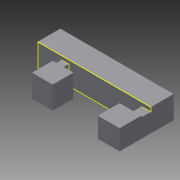
# Autodesk Inventor part: NBS(updated)
Saved by Autodesk Inventor 2013 (Build 170138000, 138)
## iProperties
Created: 2006-04-25
Part Number: NBS(updated)
Document SubType Name: Modeling
Designer: mcgratta
Material: Generic
Density: 1 g/cm^3
Author: mcgratta
Autodesk Inventor part; units mm, degrees
ref_plane "YZ Plane" through (0, 0, 0) normal (1, 0, 0) x (0, 1, 0)
ref_plane "XZ Plane" through (0, 0, 0) normal (0, 1, 0) x (-1, 0, 0)
ref_plane "XY Plane" through (0, 0, 0) normal (0, 0, 1) x (1, 0, 0)
sketch "Sketch1" plane through (0, 0, 0) normal (0, 0, 1) x (1, 0, 0)
  line L0 (-45.8384, 19.9204) -> (12144.1616, 19.9204)
  line L1 (12144.1616, 19.9204) -> (12144.1616, -2420.0796)
  line L2 (12144.1616, -2420.0796) -> (-45.8384, -2420.0796)
  line L3 (-45.8384, -2420.0796) -> (-45.8384, 19.9204)
  line L4 (12144.1616, -2420.0796) -> (11124.1616, -2420.0796)
  line L5 (11124.1616, -2420.0796) -> (11124.1616, -3450.0796)
  line L6 (11124.1616, -3450.0796) -> (12144.1616, -3450.0796)
  line L7 (12144.1616, -3450.0796) -> (12144.1616, -2420.0796)
  line L8 (12144.1616, -3450.0796) -> (9804.1616, -3450.0796)
  line L9 (9804.1616, -3450.0796) -> (9804.1616, -5790.0796)
  line L10 (9804.1616, -5790.0796) -> (12144.1616, -5790.0796)
  line L11 (12144.1616, -5790.0796) -> (12144.1616, -3450.0796)
  line L12 (2525.1057, -2420.0796) -> (3315.1057, -2420.0796)
  line L13 (3315.1057, -2420.0796) -> (3315.1057, -3360.0796)
  line L14 (3315.1057, -3360.0796) -> (2525.1057, -3360.0796)
  line L15 (2525.1057, -3360.0796) -> (2525.1057, -2420.0796)
  line L16 (2525.1057, -3360.0796) -> (4745.1057, -3360.0796)
  line L17 (4745.1057, -3360.0796) -> (4745.1057, -5600.0796)
  line L18 (4745.1057, -5600.0796) -> (2525.1057, -5600.0796)
  line L19 (2525.1057, -5600.0796) -> (2525.1057, -3360.0796)
  dimension "d0" = 12190
  dimension "d1" = 2440
  dimension "d2" = 1020
  dimension "d3" = 1030
  dimension "d4" = 2340
  dimension "d5" = 2340
  dimension "d6" = 940
  dimension "d7" = 790
  dimension "d8" = 2240
  dimension "d9" = 2220
  constraints: 40 end point, 10 parallel, 5 horizontal, 5 perpendicular, 1 point on line
  measures "d0" distance of L0.start L0.end
  measures "d1" distance of L2.end L0.start
  measures "d2" distance of L5.end L6.end
  measures "d3" distance of L6.end L1.end
  measures "d4" distance of L8.end L9.end
  measures "d5" distance of L9.end L10.end
  measures "d6" distance of L12.end L13.end
  measures "d7" distance of L13.end L14.end
  measures "d8" distance of L16.end L17.end
  measures "d9" distance of L17.end L18.end
extrude "Extrusion1" add sketch "Sketch1" along normal blind 2430 contours L14 L16 L17 L18 L19
extrude "Extrusion2" add sketch "Sketch1" along normal blind 2440 contours L0 L1 L2 L3
extrude "Extrusion3" add sketch "Sketch1" along normal blind 2000 contours L7 L6 L5 L2
extrude "Extrusion4" add sketch "Sketch1" along normal blind 2160 contours L11 L10 L9 L8 L6
extrude "Extrusion5" add sketch "Sketch1" along normal blind 2040 contours L2 L13 L14 L15
shell "Shell1" thickness 1 removed faces 0
sketch "Sketch2" plane through (-45.8384, -2420.0796, 0) normal (-1, 0, 0) x (0, 0, 1)
  line L0 (2440, 0) -> (2440, 2440) projected
  line L1 (0, 2440) -> (2440, 2440) projected
  line L2 (0, 2440) -> (0, 0) projected
  line L3 (1, 2439) -> (2439, 2439) projected
sketch "Sketch3" plane through (-45.8384, -2420.0796, 0) normal (-1, 0, 0) x (0, 0, 1)
  line L0 (0, 2440) -> (0, 0) projected
  line L1 (0, 1599) -> (2030, 1599)
  line L2 (2030, 1599) -> (2030, 839)
  line L3 (2030, 839) -> (0, 839)
  line L4 (0, 839) -> (0, 1599)
  line L5 (1, 2439) -> (2439, 2439) projected
  dimension "d25" = 2030
  dimension "d26" = 760
  dimension "d27" = 840
  constraints: 8 end point, 2 parallel, 1 horizontal, 1 perpendicular, 1 point on line
  measures "d25" distance of L1.start L1.end
  measures "d26" distance of L1.end L2.end
  measures "d27" distance between parallel lines of L1 L5
extrude "Extrusion6" cut sketch "Sketch3" against normal mid plane 2
sketch "Sketch4" plane through (-45.8384, -2420.0796, 0) normal (0, -1, 0) x (1, 0, 0)
  line L0 (2570.9442, 0) -> (2570.9442, 2040) projected
  line L1 (2570.9442, 2040) -> (3360.9442, 2040) projected
  line L2 (3360.9442, 2040) -> (3360.9442, 0) projected
  line L3 (3360.9442, 0) -> (11170, 0) projected
  line L4 (11170, 0) -> (11170, 2000) projected
  line L5 (11170, 2000) -> (12190, 2000) projected
  line L6 (12190, 2000) -> (12190, 2440) projected
  line L7 (12190, 2440) -> (0, 2440) projected
  line L8 (0, 0) -> (0, 2440) projected
  line L9 (0, 0) -> (2570.9442, 0) projected
sketch "Sketch5" plane through (9804.1616, -5790.0796, 0) normal (0, -1, 0) x (1, 0, 0)
  line L0 (0, 0) -> (0, 2160) projected
  line L1 (0, 0) -> (2340, 0) projected
  line L2 (1000, 500) -> (1340, 500)
  line L3 (1340, 500) -> (1340, 400)
  line L4 (1340, 400) -> (1000, 400)
  line L5 (1000, 400) -> (1000, 500)
  dimension "d30" = 1000
  dimension "d31" = 340
  dimension "d32" = 100
  dimension "d33" = 500
  constraints: 8 end point, 2 parallel, 1 horizontal, 1 perpendicular
  measures "d30" distance between parallel lines of L5 L0
  measures "d31" distance of L2.start L2.end
  measures "d32" distance of L2.end L3.end
  measures "d33" distance between parallel lines of L1 L2
extrude "Extrusion7" add sketch "Sketch5" against normal blind 340
sketch "Sketch6" plane through (-45.8384, 19.9204, 0) normal (0, 1, 0) x (1, 0, 0)
  line L0 (12190, 0) -> (0, 0) projected
  line L1 (11280, 0) -> (12090, 0)
  constraints: 2 end point, 1 horizontal, 1 point on line
sketch "Sketch7" plane through (-45.8384, 19.9204, 0) normal (0, 1, 0) x (1, 0, 0)
  line L0 (12190, 0) -> (12190, -2440) projected
  line L1 (12190, 0) -> (0, 0) projected
  line L2 (11280, -5) -> (12090, -5)
  line L3 (12090, -5) -> (12090, -1605)
  line L4 (12090, -1605) -> (11280, -1605)
  line L5 (11280, -1605) -> (11280, -5)
  dimension "d43" = 810
  dimension "d44" = 100
  dimension "d45" = 1600
  dimension "d46" = 1605
  constraints: 8 end point, 2 parallel, 1 horizontal, 1 perpendicular
  measures "d43" distance of L3.end L4.end
  measures "d44" distance between parallel lines of L0 L3
  measures "d45" distance of L4.end L2.start
  measures "d46" distance between parallel lines of L1 L4
extrude "Extrusion10" add sketch "Sketch7" against normal blind 2445
extrude "Extrusion11" cut sketch "Sketch7" against normal blind 2440
body "Solid1"
